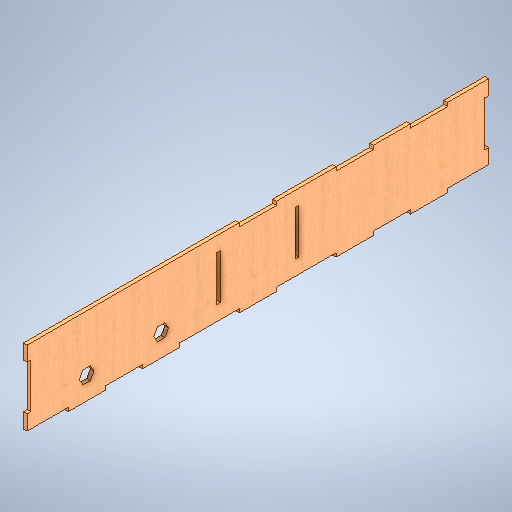
# Autodesk Inventor part: Lat3
Saved by Autodesk Inventor 2025 (Build 290162000, 162)
## iProperties
Created: 2024-11-02
Part Number: Lat3
Material: Wood (Cherry)
Document SubType Name: Sheet Metal
Designer: g.marin
Density: 0.63 g/cm^3
Sheet Metal Rule: Default
Appearance: Cherry - Natural Low Gloss
Author: g.marin
Autodesk Inventor part; units mm, degrees
ref_plane "YZ Plane" through (0, 0, 0) normal (1, 0, 0) x (0, 1, 0)
ref_plane "XZ Plane" through (0, 0, 0) normal (0, 1, 0) x (-1, 0, 0)
ref_plane "XY Plane" through (0, 0, 0) normal (0, 0, 1) x (1, 0, 0)
sketch "Sketch1" plane through (0, 0, 0) normal (1, 0, 0) x (0, 1, 0)
  line L0 (-50, 50) -> (50, 50)
  line L1 (50, 50) -> (50, -50)
  line L2 (50, -50) -> (-50, -50)
  line L3 (-50, -50) -> (-50, 50)
  line L4 (-50, 50) -> (50, -50) construction
  line L5 (50, 50) -> (-50, -50) construction
  line L6 (50, 50) -> (-50, 50)
  line L7 (-50, 50) -> (-50, 310)
  line L8 (-50, 310) -> (50, 310)
  line L9 (50, 310) -> (50, 50)
  line L10 (50, -50) -> (-50, -50)
  line L11 (-50, -50) -> (-50, -310)
  line L12 (-50, -310) -> (50, -310)
  line L13 (50, -310) -> (50, -50)
  line L14 (-50, 255) -> (-55, 255)
  line L15 (-55, 255) -> (-55, 205)
  line L16 (-55, 205) -> (-50, 205)
  line L17 (-50, 205) -> (-50, 255)
  line L18 (-50, 155) -> (-55, 155)
  line L19 (-55, 155) -> (-55, 105)
  line L20 (-55, 105) -> (-50, 105)
  line L21 (-50, 105) -> (-50, 155)
  line L22 (-50, 25) -> (-55, 25)
  line L23 (-55, 25) -> (-55, -25)
  line L24 (-55, -25) -> (-50, -25)
  line L25 (-50, -25) -> (-50, 25)
  line L26 (-50, -105) -> (-55, -105)
  line L27 (-55, -105) -> (-55, -155)
  line L28 (-55, -155) -> (-50, -155)
  line L29 (-50, -155) -> (-50, -105)
  line L30 (-50, -205) -> (-55, -205)
  line L31 (-55, -205) -> (-55, -255)
  line L32 (-55, -255) -> (-50, -255)
  line L33 (-50, -255) -> (-50, -205)
  line L34 (50, 310) -> (30, 310)
  line L35 (50, 305) -> (50, 310)
  line L36 (-50, 310) -> (-30, 310)
  line L37 (-50, 305) -> (-50, 310)
  line L38 (30, 50) -> (-30, 50)
  line L39 (-30, 50) -> (-30, 55)
  line L40 (-30, 55) -> (30, 55)
  line L41 (30, 55) -> (30, 50)
  line L42 (30, -50) -> (-21.1124, -50)
  line L43 (50, 0) -> (-50, 0) construction
  line L44 (-30, -50) -> (-30, -55)
  line L45 (-30, -55) -> (30, -55)
  line L46 (30, -55) -> (30, -50)
  line L47 (30, 310) -> (-30, 310)
  line L48 (-30, 310) -> (-30, 305)
  line L49 (-30, 305) -> (30, 305)
  line L50 (30, 305) -> (30, 310)
  line L51 (-30, -310) -> (-30, -305)
  line L52 (-30, -305) -> (30, -305)
  line L53 (30, -305) -> (30, -310)
  line L54 (50, 25) -> (45, 25)
  line L55 (45, 25) -> (45, -25)
  line L56 (45, -25) -> (50, -25)
  line L57 (50, -25) -> (50, 25)
  line L58 (50, -105) -> (45, -105)
  line L59 (45, -105) -> (45, -155)
  line L60 (45, -155) -> (50, -155)
  line L61 (50, -155) -> (50, -105)
  line L62 (50, -205) -> (45, -205)
  line L63 (45, -205) -> (45, -255)
  line L64 (45, -255) -> (50, -255)
  line L65 (50, -255) -> (50, -205)
  line L66 (-33.6603, 235) -> (-25, 240)
  line L67 (-25, 240) -> (-16.3397, 235)
  line L68 (-16.3397, 235) -> (-16.3397, 225)
  line L69 (-16.3397, 225) -> (-25, 220)
  line L70 (-25, 220) -> (-33.6603, 225)
  line L71 (-33.6603, 225) -> (-33.6603, 235)
  line L72 (-33.6603, 135) -> (-25, 140)
  line L73 (-25, 140) -> (-16.3397, 135)
  line L74 (-16.3397, 135) -> (-16.3397, 125)
  line L75 (-16.3397, 125) -> (-25, 120)
  line L76 (-25, 120) -> (-33.6603, 125)
  line L77 (-33.6603, 125) -> (-33.6603, 135)
  point P0 (0, 0)
  point P1 (-52.5, 155)
  point P2 (-52.5, 205)
  point P3 (-50, 205)
  point P4 (-50, 105)
  point P5 (-50, -155)
  point P6 (-50, -255)
  point P7 (30, -50)
  point P8 (-30, -50)
  point P9 (30, 50)
  point P10 (30, 307.5)
  point P11 (-30, -310)
  point P12 (30, 310)
  point P13 (-30, 310)
  point P14 (50, -25)
  point P15 (50, -255)
  point P16 (50, -155)
  point P17 (-25, 230)
  point P18 (-25, 130)
  dimension "d0" = 100
  dimension "d1" = 260
  dimension "d2" = 100
  dimension "d3" = 260
  dimension "d4" = 50
  dimension "d5" = 50
  dimension "d6" = 50
  dimension "d7" = 50
  dimension "d8" = 50
  dimension "d9" = 55
  dimension "d10" = 50
  dimension "d11" = 25
  dimension "d12" = 55
  dimension "d13" = 50
  dimension "d14" = 5
  dimension "d20" = 5
  dimension "d21" = 5
  dimension "d23" = 20
  dimension "d24" = 50
  dimension "d25" = 5
  dimension "d26" = 20
  dimension "d27" = 10
  dimension "d28" = 25
  dimension "d29" = 16.3397
  dimension "d30" = 25
  dimension "d31" = 10
  dimension "d32" = 25
  dimension "d33" = 16.3397
  dimension "d34" = 25
  constraints: 156 end point, 26 parallel, 17 point on line, 16 horizontal, 13 perpendicular, 9 collinear, 7 midpoint, 7 symmetric about line, 26 other
  measures "d0" distance of L11.end L12.end
  measures "d1" distance of L12.end L1.end
  measures "d2" distance of L0.end L1.end
  measures "d3" distance of L8.end L0.end
  measures "d4" distance of L14.end L15.end
  measures "d5" distance of L18.end L19.end
  measures "d6" distance of L22.end L23.end
  measures "d7" distance of L26.end L27.end
  measures "d8" distance of L30.end L31.end
  measures "d9" vertical distance of L14.end L7.end
  measures "d10" distance of point (-52.5, 155) point (-52.5, 205)
  measures "d11" vertical distance of L22.end L0.start
  measures "d12" vertical distance of L26.end L2.end
  measures "d13" distance of L30.end L27.end
  measures "d14" distance of L14.start L14.end
  measures "d20" distance between parallel lines of L0 L40
  measures "d21" distance of L49.end L34.end
  measures "d23" distance from line of point (30, 307.5) L9
  measures "d24" distance of L54.end L55.end
  measures "d25" distance between parallel lines of L55 L57
  measures "d26" distance between parallel lines of L7 L48
  measures "d27" distance of L67.end L68.end
  measures "d28" distance from line of L7 point (-25, 230)
  measures "d29" distance from line of L17 L70.end
  measures "d30" distance from line of L14 point (-25, 230)
  measures "d31" distance of L73.end L74.end
  measures "d32" distance from line of L7 point (-25, 130)
  measures "d33" distance from line of L21 L77.start
  measures "d34" distance from line of L18 point (-25, 130)
extrude "Extrusion1" add sketch "Sketch1" along normal blind 5 contours L7 L8 L48 L49 L50 L9 L0 L41 L40 L39 | L0 L1 L54 L55 L56 L2 L3 | L3 L24 L23 L22 | L20 L19 L18 L7 | L2 L44 L45 L46 L13 L58 L59 L60 L62 L63 L64 L12 L53 L52 L51 L11 | L16 L15 L14 L7 | L11 L28 L27 L26 | L11 L32 L31 L30
equation "\"BendRadius\" = Thickness"
equation "\"BendReliefWidth\" = Thickness"
equation "\"BendReliefDepth\" = 0.5 * Thickness"
equation "\"CornerReliefSize\" = 4 * Thickness"
equation "\"MinimumRemnant\" = 2 * Thickness"
equation "\"TransitionRadius\" = BendRadius"
equation "\"JacobiRadiusSize\" = BendRadius"
equation "\"GapSize\" = Thickness"
equation "\"Thickness\" = 3.048"
body "Solid1"
